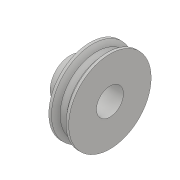
# Autodesk Inventor part: PoleaBrazos
Saved by Autodesk Inventor 2022 (Build 260153000, 153)
## iProperties
Created: 2019-11-08
Part Number: PoleaBrazos
Material: Genérico
Document SubType Name: Modeling
Designer: usuario_2
Density: 1 g/cm^3
Appearance: Valor por defecto
Author: usuario_2
Autodesk Inventor part; units mm, degrees
ref_plane "YZ Plane" through (0, 0, 0) normal (1, 0, 0) x (0, 1, 0)
ref_plane "XZ Plane" through (0, 0, 0) normal (0, 1, 0) x (-1, 0, 0)
ref_plane "XY Plane" through (0, 0, 0) normal (0, 0, 1) x (1, 0, 0)
sketch "Boceto1" plane through (0, 0, 0) normal (0, 0, 1) x (1, 0, 0)
  line L0 (-24.1261, 0) -> (26.0802, 0) construction
  line L1 (0, 10.125) -> (-30, 10.125)
  line L2 (-30, 10.125) -> (-30, 15)
  line L3 (-30, 15) -> (-15, 15)
  line L4 (-15, 15) -> (-15, 31)
  line L5 (0, 31) -> (0, 10.125)
  line L6 (-15, 31) -> (-13, 31)
  line L7 (-13, 31) -> (-10, 27.5)
  line L8 (-10, 27.5) -> (-5, 27.5)
  line L9 (-2, 31) -> (0, 31)
  line L10 (-2, 31) -> (-5, 27.5)
  line L11 (-7.5, 27.5) -> (-7.5, 0) construction
  point P0 (0, 0)
  point P1 (0, 20.5625)
  dimension "d0" = 27.5
  dimension "d1" = 31
  dimension "d2" = 10.125
  dimension "d3" = 15
  dimension "d4" = 15
  dimension "d5" = 2
  dimension "d6" = 2
  dimension "d7" = 5
  dimension "d8" = 7.5
  dimension "d9" = 15
  constraints: 24 end point, 4 perpendicular, 3 horizontal, 3 point on line, 2 midpoint, 1 parallel, 1 vertical alignment
  measures "d0" distance between parallel lines of L0 L8
  measures "d1" distance between parallel lines of L0 L9
  measures "d2" distance between parallel lines of L0 L1
  measures "d3" distance between parallel lines of L3 L0
  measures "d4" distance between parallel lines of L5 L4
  measures "d5" distance of L4.end L6.end
  measures "d6" distance of L9.start L5.start
  measures "d7" distance of L7.end L8.end
  measures "d8" distance between parallel lines of L4 L11
  measures "d9" distance of L2.end L3.end
revolve "Revolución1" add sketch "Boceto1" angle 360 about axis through (-24.1261, 0, 0) along (1, 0, 0)
sketch "Sketch2" plane through (0, 0, 0) normal (0, 0, 1) x (1, 0, 0)
  circle A0 centre (-25, 0) radius 2.25
  point P0 (0, 0)
  dimension "d11" = 4.5
  dimension "d12" = 25
  constraints: 1 centre point, 1 horizontal alignment
  measures "d11" diameter of A0
  measures "d12" distance of point (0, 0) A0.centre
extrude "Extrusion1" cut sketch "Sketch2" along normal blind 34.25
